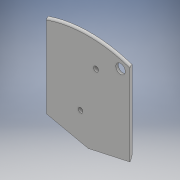
# Autodesk Inventor part: Деталь1
Saved by Autodesk Inventor 2018 (Build 220112000, 112)
## iProperties
Created: 2019-05-28
Part Number: Деталь1
Material: Типовые
Document SubType Name: Modeling
Designer: Vdalilsav
Density: 1 g/cm^3
Appearance: По умолчанию
Author: Vdalilsav
Autodesk Inventor part; units mm, degrees
ref_plane "YZ Plane" through (0, 0, 0) normal (1, 0, 0) x (0, 1, 0)
ref_plane "XZ Plane" through (0, 0, 0) normal (0, 1, 0) x (-1, 0, 0)
ref_plane "XY Plane" through (0, 0, 0) normal (0, 0, 1) x (1, 0, 0)
sketch "Эскиз1" plane through (0, 0, 0) normal (0, 1, 0) x (-1, 0, 0)
  line L0 (-34.3655, 34.8972) -> (36.1813, 34.8972) construction
  line L1 (36.1813, 34.8972) -> (36.1813, -35.6495) construction
  line L2 (36.1813, -35.6495) -> (-34.3655, -35.6495) construction
  line L3 (-34.3655, -35.6495) -> (-34.3655, 34.8972) construction
  line L4 (36.1813, 34.8972) -> (36.1813, -35.6495)
  line L5 (-34.3655, -35.6495) -> (-34.3655, 34.8972)
  arc A0 (36.1813, 34.8972) -> (-34.3655, 34.8972) centre (0.9079, -69.5429) ccw
  line L6 (-34.3655, -35.6495) -> (0.9079, -43.3385)
  line L7 (0.9079, -43.3385) -> (36.1813, -35.6495)
  point P0 (0, 0)
  constraints: 8 end point, 2 point on circle, 1 centre point, 1 parallel, 2 other
sketch "Эскиз2" plane through (0, 0, 0) normal (0, 1, 0) x (-1, 0, 0)
  circle A0 centre (-5.7378, 18.1419) radius 2.0991
  circle A1 centre (7.3616, -18.5667) radius 1.9714
  point P0 (0, 0)
  constraints: 2 centre point
sketch "Эскиз3" plane through (0, 0, 0) normal (0, 1, 0) x (-1, 0, 0)
  line L0 (1.0615, -13.152) -> (12.4155, -13.013) construction
  line L1 (12.4155, -13.013) -> (12.6378, -13.4021) construction
  line L2 (12.6378, -13.4021) -> (12.6378, -14.2498) construction
  line L3 (12.6378, -14.2498) -> (12.8046, -16.8208) construction
  line L4 (12.8046, -16.8208) -> (12.8046, -19.364) construction
  line L5 (12.8046, -19.364) -> (11.943, -20.5036) construction
  line L6 (11.943, -20.5036) -> (8.2974, -23.6186) construction
  line L7 (8.2974, -23.6186) -> (6.3443, -23.9973) construction
  line L8 (6.3443, -23.9973) -> (1.4296, -24.6519) construction
  line L9 (1.4296, -24.6519) -> (-1.1291, -24.6519) construction
  line L10 (-1.1291, -24.6519) -> (-4.5123, -23.9696) construction
  line L11 (-4.5123, -23.9696) -> (-7.5258, -22.9177) construction
  line L12 (-7.5258, -22.9177) -> (-10.1698, -21.2403) construction
  line L13 (-10.1698, -21.2403) -> (-10.8237, -19.762) construction
  line L14 (-10.8237, -19.762) -> (-10.8237, -13.152) construction
  line L15 (-10.8237, -13.152) -> (-11.097, -5.7972) construction
  line L16 (-11.097, -5.7972) -> (-10.2385, -3.0501) construction
  line L17 (-10.2385, -3.0501) -> (-9.1397, -1.8482) construction
  line L18 (-9.1397, -1.8482) -> (-7.2167, -0.921) construction
  line L19 (-7.2167, -0.921) -> (-5.4654, -0.509) construction
  line L20 (-5.4654, -0.509) -> (0, -0.509) construction
  line L21 (0, -0.509) -> (7.3775, -0.509) construction
  line L22 (7.3775, -0.509) -> (9.8661, 0) construction
  line L23 (9.8661, 0) -> (11.3908, 1.0249) construction
  line L24 (11.3908, 1.0249) -> (12.5637, 2.4715) construction
  line L25 (12.5637, 2.4715) -> (13.4629, 4.5045) construction
  line L26 (13.4629, 4.5045) -> (13.4629, 6.6743) construction
  line L27 (13.4629, 6.6743) -> (13.6819, 8.6512) construction
  line L28 (13.6819, 8.6512) -> (13.6819, 11.7226) construction
  line L29 (13.6819, 11.7226) -> (14.5006, 11.7226) construction
  line L30 (14.5006, 11.7226) -> (17.9863, 11.7226) construction
  line L31 (17.9863, 11.7226) -> (20.3437, 11.7226) construction
  line L32 (20.3437, 11.7226) -> (21.5056, 10.5811) construction
  line L33 (21.5056, 10.5811) -> (23.2284, 8.6661) construction
  line L34 (23.2284, 8.6661) -> (24.2221, 6.2455) construction
  line L35 (24.2221, 6.2455) -> (24.5024, 4.309) construction
  line L36 (24.5024, 4.309) -> (24.9865, 1.8884) construction
  line L37 (24.9865, 1.8884) -> (25.3942, -0.5577) construction
  line L38 (25.3942, -0.5577) -> (24.4374, -6.3728) construction
  line L39 (24.4374, -6.3728) -> (23.2171, -9.0779) construction
  line L40 (23.2171, -9.0779) -> (21.078, -11.3575) construction
  line L41 (21.078, -11.3575) -> (19.9903, -11.8933) construction
  line L42 (19.9903, -11.8933) -> (17.2141, -12.1531) construction
  line L43 (17.2141, -12.1531) -> (11.8565, -12.0557) construction
  line L44 (11.8565, -12.0557) -> (5.2501, -12.0557) construction
  line L45 (5.2501, -12.0557) -> (2.3472, -12.0557) construction
  line L46 (2.3472, -12.0557) -> (0.8205, -11.9623) construction
  line L47 (0.8205, -11.9623) -> (1.043, -12.7528) construction
  line L48 (1.043, -12.7528) -> (1.0615, -13.152) construction
  spline S0 degree 4 poles (1.0615, -13.152) (12.4155, -13.013) (12.6378, -13.4021) (12.6378, -14.2498) (12.8046, -16.8208) (12.8046, -19.364) (11.943, -20.5036) (8.2974, -23.6186) (6.3443, -23.9973) (1.4296, -24.6519) (-1.1291, -24.6519) (-4.5123, -23.9696) (-7.5258, -22.9177) (-10.1698, -21.2403) (-10.8237, -19.762) (-10.8237, -13.152) (-11.097, -5.7972) (-10.2385, -3.0501) (-9.1397, -1.8482) (-7.2167, -0.921) (-5.4654, -0.509) (0, -0.509) (7.3775, -0.509) (9.8661, 0) (11.3908, 1.0249) (12.5637, 2.4715) (13.4629, 4.5045) (13.4629, 6.6743) (13.6819, 8.6512) (13.6819, 11.7226) (14.5006, 11.7226) (17.9863, 11.7226) (20.3437, 11.7226) (21.5056, 10.5811) (23.2284, 8.6661) (24.2221, 6.2455) (24.5024, 4.309) (24.9865, 1.8884) (25.3942, -0.5577) (24.4374, -6.3728) (23.2171, -9.0779) (21.078, -11.3575) (19.9903, -11.8933) (17.2141, -12.1531) (11.8565, -12.0557) (5.2501, -12.0557) (2.3472, -12.0557) (0.8205, -11.9623) (1.043, -12.7528) (1.0615, -13.152) knots 1 1 1 1 1 2 3 4 5 6 7 8 9 10 11 12 13 14 15 16 17 18 19 20 21 22 23 24 25 26 27 28 29 30 31 32 33 34 35 36 37 38 39 40 41 42 43 44 45 46 47 47 47 47 47
  line L49 (0.7432, 12.8466) -> (0.6739, 11.7226) construction
  line L50 (0.6739, 11.7226) -> (-1.2578, 11.6508) construction
  line L51 (-1.2578, 11.6508) -> (-6.019, 11.7226) construction
  line L52 (-6.019, 11.7226) -> (-13.3127, 11.7226) construction
  line L53 (-13.3127, 11.7226) -> (-16.9661, 12.0459) construction
  line L54 (-16.9661, 12.0459) -> (-19.8085, 10.7887) construction
  line L55 (-19.8085, 10.7887) -> (-21.2919, 8.4504) construction
  line L56 (-21.2919, 8.4504) -> (-22.8194, 6.0427) construction
  line L57 (-22.8194, 6.0427) -> (-23.4365, 3.0987) construction
  line L58 (-23.4365, 3.0987) -> (-23.6902, -0.921) construction
  line L59 (-23.6902, -0.921) -> (-23.2567, -4.1757) construction
  line L60 (-23.2567, -4.1757) -> (-22.3068, -7.5702) construction
  line L61 (-22.3068, -7.5702) -> (-20.9562, -10.6305) construction
  line L62 (-20.9562, -10.6305) -> (-17.8496, -12.3575) construction
  line L63 (-17.8496, -12.3575) -> (-13.1471, -12.3575) construction
  line L64 (-13.1471, -12.3575) -> (-11.806, -11.6254) construction
  line L65 (-11.806, -11.6254) -> (-12.0716, -7.5319) construction
  line L66 (-12.0716, -7.5319) -> (-12.0716, -5.055) construction
  line L67 (-12.0716, -5.055) -> (-11.1905, -3.2812) construction
  line L68 (-11.1905, -3.2812) -> (-9.9658, -1.5679) construction
  line L69 (-9.9658, -1.5679) -> (-7.4334, 0) construction
  line L70 (-7.4334, 0) -> (-6.341, 0.6654) construction
  line L71 (-6.341, 0.6654) -> (6.7385, 0.6654) construction
  line L72 (6.7385, 0.6654) -> (9.0693, 0.8835) construction
  line L73 (9.0693, 0.8835) -> (10.963, 2.174) construction
  line L74 (10.963, 2.174) -> (12.055, 3.9119) construction
  line L75 (12.055, 3.9119) -> (12.7212, 9.512) construction
  line L76 (12.7212, 9.512) -> (12.3738, 12.8466) construction
  line L77 (12.3738, 12.8466) -> (12.3738, 18.5043) construction
  line L78 (12.3738, 18.5043) -> (11.9483, 20.7651) construction
  line L79 (11.9483, 20.7651) -> (10.0542, 22.5664) construction
  line L80 (10.0542, 22.5664) -> (7.8959, 23.3034) construction
  line L81 (7.8959, 23.3034) -> (5.1755, 23.8166) construction
  line L82 (5.1755, 23.8166) -> (1.9586, 23.9915) construction
  line L83 (1.9586, 23.9915) -> (-2.0367, 23.9915) construction
  line L84 (-2.0367, 23.9915) -> (-5.1578, 23.2571) construction
  line L85 (-5.1578, 23.2571) -> (-8.6217, 22.4421) construction
  line L86 (-8.6217, 22.4421) -> (-10.7436, 20.9652) construction
  line L87 (-10.7436, 20.9652) -> (-11.1729, 18.7628) construction
  line L88 (-11.1729, 18.7628) -> (-11.1729, 15.2971) construction
  line L89 (-11.1729, 15.2971) -> (-11.0362, 12.806) construction
  line L90 (-11.0362, 12.806) -> (-7.6017, 12.806) construction
  line L91 (-7.6017, 12.806) -> (-3.0076, 12.806) construction
  line L92 (-3.0076, 12.806) -> (-1.0737, 12.806) construction
  line L93 (-1.0737, 12.806) -> (0.7432, 12.8466) construction
  spline S1 degree 4 poles (0.7432, 12.8466) (0.6739, 11.7226) (-1.2578, 11.6508) (-6.019, 11.7226) (-13.3127, 11.7226) (-16.9661, 12.0459) (-19.8085, 10.7887) (-21.2919, 8.4504) (-22.8194, 6.0427) (-23.4365, 3.0987) (-23.6902, -0.921) (-23.2567, -4.1757) (-22.3068, -7.5702) (-20.9562, -10.6305) (-17.8496, -12.3575) (-13.1471, -12.3575) (-11.806, -11.6254) (-12.0716, -7.5319) (-12.0716, -5.055) (-11.1905, -3.2812) (-9.9658, -1.5679) (-7.4334, 0) (-6.341, 0.6654) (6.7385, 0.6654) (9.0693, 0.8835) (10.963, 2.174) (12.055, 3.9119) (12.7212, 9.512) (12.3738, 12.8466) (12.3738, 18.5043) (11.9483, 20.7651) (10.0542, 22.5664) (7.8959, 23.3034) (5.1755, 23.8166) (1.9586, 23.9915) (-2.0367, 23.9915) (-5.1578, 23.2571) (-8.6217, 22.4421) (-10.7436, 20.9652) (-11.1729, 18.7628) (-11.1729, 15.2971) (-11.0362, 12.806) (-7.6017, 12.806) (-3.0076, 12.806) (-1.0737, 12.806) (0.7432, 12.8466) knots 1 1 1 1 1 2 3 4 5 6 7 8 9 10 11 12 13 14 15 16 17 18 19 20 21 22 23 24 25 26 27 28 29 30 31 32 33 34 35 36 37 38 39 40 41 42 43 43 43 43 43
  point P0 (0, 0)
  constraints: 12 horizontal, 6 vertical, 3 parallel, 2 perpendicular, 3 other
extrude "Выдавливание1" add sketch "Эскиз1" against normal blind 2
sketch "Эскиз4" plane through (0, 0, 0) normal (0, 1, 0) x (1, 0, 0)
  line L0 (34.3655, 35.6495) -> (34.3655, -34.8972) projected
  circle A0 centre (26.4343, -28.5977) radius 4
  point P0 (0, 0)
  dimension "d19" = 8
  constraints: 1 centre point
  measures "d19" diameter of A0
extrude "Выдавливание2" cut sketch "Эскиз4" against normal blind 2
extrude "Выдавливание3" add sketch "Эскиз3" along normal blind 1
extrude "Выдавливание4" cut sketch "Эскиз2" along normal mid plane 4
fillet "Сопряжение1" radius 1.75 2 edges at (-0.9079, -2, 40.693) (-0.9079, 0, 40.693)
fillet "Сопряжение2" radius 10.5 2 edges at (16.7288, 0, -39.494) (-18.5446, 0, -39.494)
